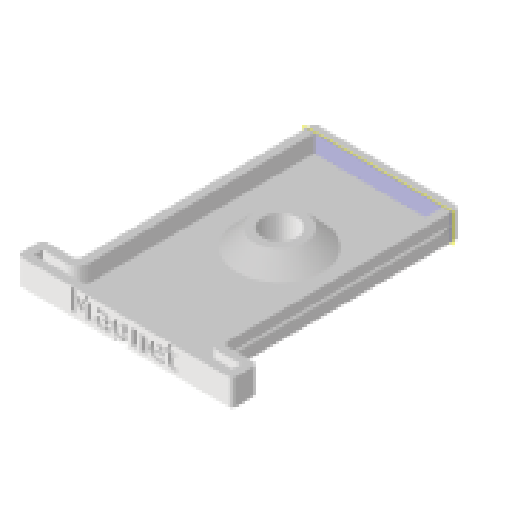
# Autodesk Inventor part: 00_Slider_4_magnet_tshirt
Saved by Autodesk Inventor 2025.1 (Build 291241020, 241B)
## iProperties
Created: 2021-10-22
Part Number: 00_Slider_4_magnet_tshirt
Material: Generic
Document SubType Name: Modeling
Designer: diederichbenedict
Density: 1 g/cm^3
Appearance: Default
Author: diederichbenedict
Autodesk Inventor part; units mm, degrees
ref_plane "YZ Plane" through (0, 0, 0) normal (1, 0, 0) x (0, 1, 0)
ref_plane "XZ Plane" through (0, 0, 0) normal (0, 1, 0) x (-1, 0, 0)
ref_plane "XY Plane" through (0, 0, 0) normal (0, 0, 1) x (1, 0, 0)
sketch "Sketch1" plane through (0, 0, 0) normal (0, 1, 0) x (-1, 0, 0)
  line L0 (-16.92, 27.5) -> (16.92, 27.5)
  line L1 (16.92, 27.5) -> (16.92, -27.5)
  line L2 (16.92, -27.5) -> (-16.92, -27.5)
  line L3 (-16.92, -27.5) -> (-16.92, 27.5)
  line L4 (-16.92, 27.5) -> (16.92, -27.5) construction
  line L5 (16.92, 27.5) -> (-16.92, -27.5) construction
  line L6 (-25, 33.5) -> (25, 33.5)
  line L7 (25, 33.5) -> (25, 27.5)
  line L8 (25, 27.5) -> (-25, 27.5)
  line L9 (-25, 27.5) -> (-25, 33.5)
  line L10 (-25, 33.5) -> (25, 27.5) construction
  line L11 (25, 33.5) -> (-25, 27.5) construction
  circle A0 centre (0, -2.5) radius 4
  point P0 (0, 0)
  point P1 (0, 30.5)
  point P2 (0, 27.5)
  dimension "d0" = 33.84
  dimension "d1" = 55
  dimension "d3" = 50
  dimension "d4" = 6
  dimension "d14" = 8
  dimension "d15" = 25
  constraints: 24 end point, 6 midpoint, 4 parallel, 2 horizontal, 2 perpendicular, 1 centre point
  measures "d0" distance of L1.end L2.end
  measures "d1" distance of L0.end L1.end
  measures "d3" distance of L7.end L8.end
  measures "d4" distance of L6.end L7.end
  measures "d14" diameter of A0
  measures "d15" distance from line of A0.centre L2
extrude "Extrusion1" add sketch "Sketch1" along normal blind 6
fillet "Fillet1" radius 1 8 edges at (25, 3, 33.5) (25, 3, 27.5) (-25, 3, 33.5) (-25, 3, 27.5) (-16.92, 3, 27.5) (-16.92, 3, -27.5) (16.92, 3, -27.5) (16.92, 3, 27.5)
shell "Shell1" thickness 2 removed faces 1 at (0.1607, 6, 18.1569)
sketch "Sketch3" plane through (0, 6, 33.5) normal (0, 0, 1) x (1, 0, 0)
  line L0 (-12.975, -0.1925) -> (12.2508, -0.1925) construction
  line L1 (12.2508, -0.1925) -> (12.2508, -5.3797) construction
  line L2 (12.2508, -5.3797) -> (-12.975, -5.3797) construction
  line L3 (-12.975, -5.3797) -> (-12.975, -0.1925) construction
  line L4 (-7.4973, -5.0625) -> (-8.7128, -5.0625)
  line L5 (-8.7128, -5.0625) -> (-8.7128, -1.8342)
  line L6 (-8.7128, -1.8342) -> (-9.5968, -3.918)
  line L7 (-9.5968, -3.918) -> (-10.4335, -3.918)
  line L8 (-10.4335, -3.918) -> (-11.3175, -1.8342)
  line L9 (-11.3175, -1.8342) -> (-11.3175, -5.0625)
  line L10 (-11.3175, -5.0625) -> (-12.4699, -5.0625)
  line L11 (-12.4699, -5.0625) -> (-12.4699, -0.1925)
  line L12 (-12.4699, -0.1925) -> (-11.061, -0.1925)
  line L13 (-11.061, -0.1925) -> (-9.9796, -2.5959)
  line L14 (-9.9796, -2.5959) -> (-8.9062, -0.1925)
  line L15 (-8.9062, -0.1925) -> (-7.4973, -0.1925)
  line L16 (-7.4973, -0.1925) -> (-7.4973, -5.0625)
  spline S0 degree 2 poles (-4.5295, -4.6718) (-4.6479, -4.7704) (-4.8334, -4.9283) (-4.9912, -5.0072) knots 0 0 0 1 2 2 2
  spline S1 degree 2 poles (-4.9912, -5.0072) (-5.1451, -5.0822) (-5.4372, -5.1611) (-5.6976, -5.1611) knots 0 0 0 1 2 2 2
  spline S2 degree 2 poles (-5.6976, -5.1611) (-6.187, -5.1611) (-6.8303, -4.506) (-6.8303, -4.0088) knots 0 0 0 1 2 2 2
  spline S3 degree 2 poles (-6.8303, -4.0088) (-6.8303, -3.6023) (-6.5027, -3.0971) (-6.1949, -2.9511) knots 0 0 0 1 2 2 2
  spline S4 degree 2 poles (-6.1949, -2.9511) (-5.8831, -2.8011) (-5.0188, -2.6827) (-4.5216, -2.6512) knots 0 0 0 1 2 2 2
  line L17 (-4.5216, -2.6512) -> (-4.5216, -2.6314)
  spline S5 degree 2 poles (-4.5216, -2.6314) (-4.5216, -2.3275) (-4.9715, -2.0947) (-5.4214, -2.0947) knots 0 0 0 1 2 2 2
  spline S6 degree 2 poles (-5.4214, -2.0947) (-5.6227, -2.0947) (-6.1673, -2.2407) (-6.4238, -2.3552) knots 0 0 0 1 2 2 2
  line L18 (-6.4238, -2.3552) -> (-6.5225, -2.3552)
  line L19 (-6.5225, -2.3552) -> (-6.5225, -1.4672)
  spline S7 degree 2 poles (-6.5225, -1.4672) (-6.3528, -1.4198) (-5.595, -1.2857) (-5.2083, -1.2857) knots 0 0 0 1 2 2 2
  spline S8 degree 2 poles (-5.2083, -1.2857) (-4.2611, -1.2857) (-3.3929, -1.9171) (-3.3929, -2.5643) knots 0 0 0 1 2 2 2
  line L20 (-3.3929, -2.5643) -> (-3.3929, -5.0625)
  line L21 (-3.3929, -5.0625) -> (-4.5295, -5.0625)
  line L22 (-4.5295, -5.0625) -> (-4.5295, -4.6718)
  line L23 (-4.5295, -4.1035) -> (-4.5295, -3.3418)
  spline S9 degree 2 poles (-4.5295, -3.3418) (-4.8215, -3.3694) (-5.1806, -3.4128) (-5.3543, -3.476) knots 0 0 0 1 2 2 2
  spline S10 degree 2 poles (-5.3543, -3.476) (-5.5082, -3.5273) (-5.674, -3.7404) (-5.674, -3.914) knots 0 0 0 1 2 2 2
  spline S11 degree 2 poles (-5.674, -3.914) (-5.674, -4.1706) (-5.3938, -4.3639) (-5.1214, -4.3639) knots 0 0 0 1 2 2 2
  spline S12 degree 2 poles (-5.1214, -4.3639) (-4.9715, -4.3639) (-4.6558, -4.2258) (-4.5295, -4.1035) knots 0 0 0 1 2 2 2
  spline S13 degree 2 poles (0.7944, -4.6402) (0.7944, -5.1493) (0.4984, -5.8636) (0.2458, -6.061) knots 0 0 0 1 2 2 2
  spline S14 degree 2 poles (0.2458, -6.061) (-0.0107, -6.2622) (-0.7211, -6.4438) (-1.1552, -6.4438) knots 0 0 0 1 2 2 2
  spline S15 degree 2 poles (-1.1552, -6.4438) (-1.5222, -6.4438) (-2.1813, -6.349) (-2.422, -6.2859) knots 0 0 0 1 2 2 2
  line L24 (-2.422, -6.2859) -> (-2.422, -5.3664)
  line L25 (-2.422, -5.3664) -> (-2.2879, -5.3664)
  spline S16 degree 2 poles (-2.2879, -5.3664) (-2.205, -5.3979) (-1.9721, -5.4769) (-1.8537, -5.5084) knots 0 0 0 1 2 2 2
  spline S17 degree 2 poles (-1.8537, -5.5084) (-1.7117, -5.544) (-1.4433, -5.5913) (-1.3052, -5.5913) knots 0 0 0 1 2 2 2
  spline S18 degree 2 poles (-1.3052, -5.5913) (-1.0131, -5.5913) (-0.6264, -5.4729) (-0.5277, -5.3624) knots 0 0 0 1 2 2 2
  spline S19 degree 2 poles (-0.5277, -5.3624) (-0.429, -5.248) (-0.3501, -4.9401) (-0.3501, -4.7033) knots 0 0 0 1 2 2 2
  line L26 (-0.3501, -4.7033) -> (-0.3501, -4.6363)
  spline S20 degree 2 poles (-0.3501, -4.6363) (-0.5435, -4.806) (-1.0486, -5.0112) (-1.317, -5.0112) knots 0 0 0 1 2 2 2
  spline S21 degree 2 poles (-1.317, -5.0112) (-2.0313, -5.0112) (-2.8048, -4.0837) (-2.8048, -3.1326) knots 0 0 0 1 2 2 2
  spline S22 degree 2 poles (-2.8048, -3.1326) (-2.8048, -2.7025) (-2.5681, -2.0158) (-2.3549, -1.775) knots 0 0 0 1 2 2 2
  spline S23 degree 2 poles (-2.3549, -1.775) (-2.1497, -1.5422) (-1.5775, -1.2896) (-1.2657, -1.2896) knots 0 0 0 1 2 2 2
  spline S24 degree 2 poles (-1.2657, -1.2896) (-0.9855, -1.2896) (-0.5395, -1.4317) (-0.358, -1.5501) knots 0 0 0 1 2 2 2
  line L27 (-0.358, -1.5501) -> (-0.3146, -1.3883)
  line L28 (-0.3146, -1.3883) -> (0.7944, -1.3883)
  line L29 (0.7944, -1.3883) -> (0.7944, -4.6402)
  line L30 (-0.3501, -3.9062) -> (-0.3501, -2.2407)
  spline S25 degree 2 poles (-0.3501, -2.2407) (-0.433, -2.2013) (-0.6816, -2.15) (-0.8079, -2.15) knots 0 0 0 1 2 2 2
  spline S26 degree 2 poles (-0.8079, -2.15) (-1.2183, -2.15) (-1.6327, -2.6827) (-1.6327, -3.1603) knots 0 0 0 1 2 2 2
  spline S27 degree 2 poles (-1.6327, -3.1603) (-1.6327, -3.3971) (-1.5696, -3.7286) (-1.4867, -3.8548) knots 0 0 0 1 2 2 2
  spline S28 degree 2 poles (-1.4867, -3.8548) (-1.4038, -3.9811) (-1.1394, -4.1074) (-0.9342, -4.1074) knots 0 0 0 1 2 2 2
  spline S29 degree 2 poles (-0.9342, -4.1074) (-0.7803, -4.1074) (-0.4843, -4.0009) (-0.3501, -3.9062) knots 0 0 0 1 2 2 2
  line L31 (5.1079, -5.0625) -> (3.9555, -5.0625)
  line L32 (3.9555, -5.0625) -> (3.9555, -3.2431)
  spline S30 degree 2 poles (3.9555, -3.2431) (3.9555, -3.0182) (3.92, -2.5762) (3.8727, -2.4736) knots 0 0 0 1 2 2 2
  spline S31 degree 2 poles (3.8727, -2.4736) (3.8135, -2.3473) (3.5925, -2.2407) (3.403, -2.2407) knots 0 0 0 1 2 2 2
  spline S32 degree 2 poles (3.403, -2.2407) (3.2649, -2.2407) (2.9768, -2.3473) (2.815, -2.4617) knots 0 0 0 1 2 2 2
  line L33 (2.815, -2.4617) -> (2.815, -5.0625)
  line L34 (2.815, -5.0625) -> (1.6705, -5.0625)
  line L35 (1.6705, -5.0625) -> (1.6705, -1.3883)
  line L36 (1.6705, -1.3883) -> (2.815, -1.3883)
  line L37 (2.815, -1.3883) -> (2.815, -1.7948)
  spline S33 degree 2 poles (2.815, -1.7948) (3.0952, -1.558) (3.628, -1.2896) (3.9516, -1.2896) knots 0 0 0 1 2 2 2
  spline S34 degree 2 poles (3.9516, -1.2896) (4.512, -1.2896) (5.1079, -2) (5.1079, -2.6709) knots 0 0 0 1 2 2 2
  line L38 (5.1079, -2.6709) -> (5.1079, -5.0625)
  spline S35 degree 2 poles (7.8389, -5.1611) (6.797, -5.1611) (5.6881, -4.1666) (5.6881, -3.2471) knots 0 0 0 1 2 2 2
  spline S36 degree 2 poles (5.6881, -3.2471) (5.6881, -2.3473) (6.722, -1.2738) (7.6534, -1.2738) knots 0 0 0 1 2 2 2
  spline S37 degree 2 poles (7.6534, -1.2738) (8.494, -1.2738) (9.3465, -2.1855) (9.3465, -3.03) knots 0 0 0 1 2 2 2
  line L39 (9.3465, -3.03) -> (9.3465, -3.4444)
  line L40 (9.3465, -3.4444) -> (6.8325, -3.4444)
  spline S38 degree 2 poles (6.8325, -3.4444) (6.8483, -3.7009) (7.0338, -4.0403) (7.1838, -4.1429) knots 0 0 0 1 2 2 2
  spline S39 degree 2 poles (7.1838, -4.1429) (7.3298, -4.2456) (7.7245, -4.3324) (7.9573, -4.3324) knots 0 0 0 1 2 2 2
  spline S40 degree 2 poles (7.9573, -4.3324) (8.1546, -4.3324) (8.5414, -4.2456) (8.7032, -4.1706) knots 0 0 0 1 2 2 2
  spline S41 degree 2 poles (8.7032, -4.1706) (8.8453, -4.1114) (9.0821, -3.9654) (9.157, -3.9101) knots 0 0 0 1 2 2 2
  line L41 (9.157, -3.9101) -> (9.2794, -3.9101)
  line L42 (9.2794, -3.9101) -> (9.2794, -4.8573)
  spline S42 degree 2 poles (9.2794, -4.8573) (9.1373, -4.9125) (8.9084, -5.0072) (8.7032, -5.0546) knots 0 0 0 1 2 2 2
  spline S43 degree 2 poles (8.7032, -5.0546) (8.5177, -5.1059) (8.1231, -5.1611) (7.8389, -5.1611) knots 0 0 0 1 2 2 2
  spline S44 degree 2 poles (8.2178, -2.7538) (8.2099, -2.3907) (7.8902, -2.0079) (7.5627, -2.0079) knots 0 0 0 1 2 2 2
  spline S45 degree 2 poles (7.5627, -2.0079) (7.2272, -2.0079) (6.8483, -2.4104) (6.8286, -2.7538) knots 0 0 0 1 2 2 2
  line L43 (6.8286, -2.7538) -> (8.2178, -2.7538)
  spline S46 degree 2 poles (11.3395, -5.1335) (10.6409, -5.1335) (10.0016, -4.5573) (10.0016, -3.9022) knots 0 0 0 1 2 2 2
  line L44 (10.0016, -3.9022) -> (10.0016, -2.1855)
  line L45 (10.0016, -2.1855) -> (9.5635, -2.1855)
  line L46 (9.5635, -2.1855) -> (9.5635, -1.3883)
  line L47 (9.5635, -1.3883) -> (10.0016, -1.3883)
  line L48 (10.0016, -1.3883) -> (10.0016, -0.3385)
  line L49 (10.0016, -0.3385) -> (11.1461, -0.3385)
  line L50 (11.1461, -0.3385) -> (11.1461, -1.3883)
  line L51 (11.1461, -1.3883) -> (12.2511, -1.3883)
  line L52 (12.2511, -1.3883) -> (12.2511, -2.1855)
  line L53 (12.2511, -2.1855) -> (11.1461, -2.1855)
  line L54 (11.1461, -2.1855) -> (11.1461, -3.4918)
  spline S47 degree 2 poles (11.1461, -3.4918) (11.1461, -3.6851) (11.154, -3.9732) (11.2013, -4.0877) knots 0 0 0 1 2 2 2
  spline S48 degree 2 poles (11.2013, -4.0877) (11.2487, -4.2021) (11.4815, -4.3363) (11.7025, -4.3363) knots 0 0 0 1 2 2 2
  spline S49 degree 2 poles (11.7025, -4.3363) (11.7973, -4.3363) (12.0933, -4.2574) (12.1524, -4.2258) knots 0 0 0 1 2 2 2
  line L55 (12.1524, -4.2258) -> (12.2511, -4.2258)
  line L56 (12.2511, -4.2258) -> (12.2511, -5.0309)
  spline S50 degree 2 poles (12.2511, -5.0309) (12.0656, -5.0783) (11.6473, -5.1335) (11.3395, -5.1335) knots 0 0 0 1 2 2 2
  point P0 (0, -6)
  constraints: 2 other
extrude "Extrusion3" cut sketch "Sketch3" against normal blind 1
chamfer "Chamfer1" distance 4 angle 45 1 edges at (6, 2, -2.5)
ref_plane "Work Plane1" through (15.92, 0, -25.5) normal (0, 0, -1) x (-1, 0, 0)
sketch "Sketch4" plane through (15.92, 0, -25.5) normal (0, 0, -1) x (-1, 0, 0)
  line L0 (-1, 6) -> (-1, 0) projected
  line L1 (32.84, 0) -> (32.84, 6) projected
  circle A0 centre (-1, 3) radius 0.5
  circle A1 centre (32.84, 3) radius 0.5
  point P0 (15.92, 0)
  dimension "d21" = 1
  dimension "d22" = 1
  constraints: 2 centre point, 2 midpoint
  measures "d21" diameter of A0
  measures "d22" diameter of A1
extrude "Extrusion4" add sketch "Sketch4" against normal up to surface (53 mm away)
sketch "Sketch5" plane through (0, 6, 0) normal (0, 1, 0) x (1, 0, 0)
  line L0 (16.92, -26.5) -> (16.92, 25.5) projected
  line L1 (16.92, 25.5) -> (16.92, -26.5) projected
  line L2 (16.92, 25.5) -> (16.92, 25.5) projected
  line L3 (-16.92, -26.5) -> (-16.92, 25.5) projected
  line L4 (-16.92, 25.5) -> (-16.92, -26.5) projected
  line L5 (-16.92, 25.5) -> (-16.92, 25.5) projected
  line L6 (16.92, 25.5) -> (17.9482, 19.669)
  line L7 (16.92, 25.5) -> (22.841, 25.5) construction
  line L8 (17.9482, 19.669) -> (19.2579, 29.9926)
  line L9 (19.2579, 29.9926) -> (16.92, 25.5)
  line L10 (-16.92, 25.5) -> (-18.7778, 20.3956)
  line L11 (-16.92, 25.5) -> (-11.4881, 25.5) construction
  line L12 (-18.7778, 20.3956) -> (-20.4331, 29.7833)
  line L13 (-20.4331, 29.7833) -> (-16.92, 25.0895)
  line L14 (-16.92, 26.5) -> (-16.92, -26.5) projected
  point P0 (0, 0)
  point P1 (-17.0205, 25.2238)
  dimension "d25" = 80
  dimension "d26" = 110
  constraints: 16 end point, 2 equal length, 2 horizontal, 1 parallel, 1 point on line
  measures "d25" angle of L6 L7
  measures "d26" angle of L10 L11
extrude "Extrusion5" cut sketch "Sketch5" against normal blind 10 contours L10 L12 L13 | L9 L8 L6
body "Solid1"
